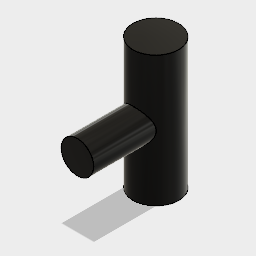
bearingv1 (Autodesk Fusion 360 design; units mm, degrees)
Autodesk Fusion 360 part; units mm, degrees
sketch "スケッチ1" plane through (0, 0, 0) normal (0, 1, 0) x (1, 0, 0)
  line L0 (0, 5) -> (0, 5)
  line L1 (1.75, 0) -> (22.5, 0)
  line L2 (1.75, 0) -> (22.5, 0)
  line L3 (0, -1.75) -> (0, -22.5)
  circle A0 centre (0, 0) radius 3.5
  dimension "d35" = 7
  measures "d35" diameter of A0
extrude "押し出し5" add sketch "スケッチ1" along normal mid plane 20
sketch "スケッチ11" plane through (0, 0, 0) normal (0, 1, 0) x (1, 0, 0)
  line L0 (-2.5, 0) -> (0, 0)
  line L1 (0, 0) -> (0, -12)
  line L2 (0, -12) -> (-2.5, -12)
  line L3 (-2.5, -12) -> (-2.5, 0)
  line L4 (0, -1.75) -> (0, -22.5)
  dimension "d38" = 2.5
  dimension "d39" = 12
  measures "d38" distance of L0.start L0.end
  measures "d39" distance of L0.start L2.end
revolve "回転1" add sketch "スケッチ11" angle 360 about axis through (0, 0, 0) along (0, 0, 1)
extrude "押し出し3" [suppressed]
